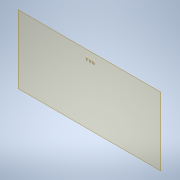
# Autodesk Inventor part: tss logo
Saved by Autodesk Inventor 2020 (Build 240168000, 168)
## iProperties
Created: 2020-06-11
Part Number: tss logo
Material: ABS Plastic
Document SubType Name: Modeling
Designer: Gebruiker
Density: 1.06 g/cm^3
Appearance: Smooth - White
Author: Gebruiker
Autodesk Inventor part; units mm, degrees
ref_plane "YZ Plane" through (0, 0, 0) normal (1, 0, 0) x (0, 1, 0)
ref_plane "XZ Plane" through (0, 0, 0) normal (0, 1, 0) x (-1, 0, 0)
ref_plane "Work Plane1" through (0, 0, 0) normal (0, 0, 1) x (1, 0, 0)
sketch "Sketch1" plane through (0, 0, 0) normal (0, 0, 1) x (1, 0, 0)
  circle A0 centre (-95.35, -29.81) radius 5 projected
  circle A1 centre (-95.35, 29.81) radius 4.15 projected
  circle A2 centre (75.35, -29.81) radius 4.15 projected
  circle A3 centre (75.35, 9.93) radius 4.15 projected
  circle A4 centre (95.35, 29.81) radius 4.15 projected
  circle A5 centre (95.35, -9.93) radius 4.15 projected
  circle A6 centre (-95.35, -9.93) radius 4.15 projected
  circle A7 centre (-75.35, 9.93) radius 4.15 projected
  circle A8 centre (-75.35, 29.81) radius 4.15 projected
  circle A9 centre (-75.35, -29.81) radius 4.15 projected
  circle A10 centre (95.35, -29.81) radius 4.15 projected
  circle A11 centre (95.35, 9.93) radius 4.15 projected
  circle A12 centre (75.35, 29.81) radius 4.15 projected
  circle A13 centre (75.35, -9.93) radius 4.15 projected
  circle A14 centre (-75.35, -9.93) radius 4.15 projected
  circle A15 centre (-95.35, 9.93) radius 4.15 projected
  line L0 (-53, 34) -> (53, 34) projected
  line L1 (53, 34) -> (53, -34) projected
  line L2 (53, -34) -> (-53, -34) projected
  line L3 (-53, -34) -> (-53, 34) projected
  line L4 (0, 46.4465) -> (0, 46.1965) projected
  line L5 (0, 46.1965) -> (2.9831, 46.1965) projected
  line L6 (2.9831, 46.1965) -> (2.9831, 44.6965) projected
  line L7 (2.9831, 44.6965) -> (-1.0169, 44.6965) projected
  line L8 (-1.0169, 44.6965) -> (-1.0169, 47.9465) projected
  line L9 (-1.0169, 47.9465) -> (2.9831, 47.9465) projected
  line L10 (2.9831, 47.9465) -> (2.9831, 46.4465) projected
  line L11 (2.9831, 46.4465) -> (0, 46.4465) projected
  line L12 (4.5797, 46.4465) -> (4.5797, 47.9465) projected
  line L13 (4.5797, 47.9465) -> (8.5797, 47.9465) projected
  line L14 (8.5797, 47.9465) -> (8.5797, 46.4465) projected
  line L15 (8.5797, 46.4465) -> (4.5797, 46.4465) projected
  line L16 (2.9831, 44.4465) -> (2.9831, 42.9465) projected
  line L17 (2.9831, 42.9465) -> (-1.0169, 42.9465) projected
  line L18 (-1.0169, 42.9465) -> (-1.0169, 44.4465) projected
  line L19 (-1.0169, 44.4465) -> (2.9831, 44.4465) projected
  line L20 (7.5636, 44.4465) -> (7.5636, 44.6965) projected
  line L21 (7.5636, 44.6965) -> (4.5797, 44.6965) projected
  line L22 (4.5797, 44.6965) -> (4.5797, 46.1965) projected
  line L23 (4.5797, 46.1965) -> (8.5797, 46.1965) projected
  line L24 (8.5797, 46.1965) -> (8.5797, 42.9465) projected
  line L25 (8.5797, 42.9465) -> (4.5797, 42.9465) projected
  line L26 (4.5797, 42.9465) -> (4.5797, 44.4465) projected
  line L27 (4.5797, 44.4465) -> (7.5636, 44.4465) projected
  line L28 (-2.942, 47.9465) -> (-2.942, 45.9465) projected
  line L29 (-2.942, 45.9465) -> (-3.942, 45.9465) projected
  line L30 (-3.942, 45.9465) -> (-3.942, 42.9465) projected
  line L31 (-3.942, 42.9465) -> (-5.942, 42.9465) projected
  line L32 (-5.942, 42.9465) -> (-5.942, 45.9465) projected
  line L33 (-5.942, 45.9465) -> (-6.942, 45.9465) projected
  line L34 (-6.942, 45.9465) -> (-6.942, 47.9465) projected
  line L35 (-6.942, 47.9465) -> (-2.942, 47.9465) projected
  arc A16 (-69.3301, 52.5) -> (-73.6603, 55) centre (-73.6603, 50) ccw projected
  line L36 (-73.6603, 55) -> (-110, 55) projected
  arc A17 (-110, 55) -> (-115, 50) centre (-110, 50) ccw projected
  line L37 (-115, 50) -> (-115, -50) projected
  arc A18 (-115, -50) -> (-110, -55) centre (-110, -50) ccw projected
  line L38 (-110, -55) -> (-73.6603, -55) projected
  arc A19 (-73.6603, -55) -> (-69.3301, -52.5) centre (-73.6603, -50) ccw projected
  arc A20 (-65, -50) -> (-69.3301, -52.5) centre (-65, -55) ccw projected
  line L39 (-65, -50) -> (65, -50) projected
  arc A21 (69.3301, -52.5) -> (65, -50) centre (65, -55) ccw projected
  arc A22 (69.3301, -52.5) -> (73.6603, -55) centre (73.6603, -50) ccw projected
  line L40 (73.6603, -55) -> (110, -55) projected
  arc A23 (110, -55) -> (115, -50) centre (110, -50) ccw projected
  line L41 (115, -50) -> (115, 50) projected
  arc A24 (115, 50) -> (110, 55) centre (110, 50) ccw projected
  line L42 (110, 55) -> (73.6603, 55) projected
  arc A25 (73.6603, 55) -> (69.3301, 52.5) centre (73.6603, 50) ccw projected
  arc A26 (65, 50) -> (69.3301, 52.5) centre (65, 55) ccw projected
  line L43 (65, 50) -> (-65, 50) projected
  arc A27 (-69.3301, 52.5) -> (-65, 50) centre (-65, 55) ccw projected
  point P0 (0, 0)
extrude "Extrusion1" add sketch "Sketch1" against normal blind 2 contours L4 L5 L6 L7 L8 L9 L10 L11 | L12 L13 L14 L15 | L16 L17 L18 L19 | L20 L21 L22 L23 L24 L25 L26 L27 | L28 L29 L30 L31 L32 L33 L34 L35
body "Solid1"
